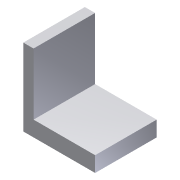
# Autodesk Inventor part: Rib support
Saved by Autodesk Inventor 2011 (Build 150239000, 239)
## iProperties
Created: 2005-07-15
Part Number: Rib support
Document SubType Name: Modeling
Designer: Administrator
Manufacturer: Standard
Standards Organization: Custom
Density: 1 g/cm^3
Author: Administrator
Autodesk Inventor part; units mm, degrees
ref_plane "YZ Plane" through (0, 0, 0) normal (1, 0, 0) x (0, 1, 0)
ref_plane "XZ Plane" through (0, 0, 0) normal (0, 1, 0) x (-1, 0, 0)
ref_plane "XY Plane" through (0, 0, 0) normal (0, 0, 1) x (1, 0, 0)
sketch "Sketch1" plane through (0, 0, 0) normal (0, 0, 1) x (1, 0, 0)
  line L0 (-38.1, 25.4) -> (-38.1, -22.225)
  line L1 (-38.1, -22.225) -> (6.35, -22.225)
  line L2 (6.35, -22.225) -> (6.35, -12.7)
  line L3 (6.35, -12.7) -> (-31.75, -12.7)
  line L4 (-31.75, -12.7) -> (-31.75, 25.4)
  line L5 (-31.75, 25.4) -> (-38.1, 25.4)
  constraints: 12 end point, 4 parallel, 1 perpendicular
extrude "Extrusion1" add sketch "Sketch1" along normal blind 38.1
body "Solid1"
